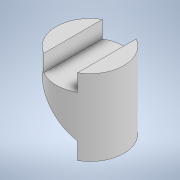
# Autodesk Inventor part: Деталь1вар2
Saved by Autodesk Inventor 2021.1 (Build 251245010, 245A)
## iProperties
Created: 2023-10-25
Part Number: Деталь1вар2
Material: Типовые
Document SubType Name: Modeling
Designer: Lenovo
Density: 1 g/cm^3
Appearance: По умолчанию
Author: Lenovo
Autodesk Inventor part; units mm, degrees
ref_plane "YZ Plane" through (0, 0, 0) normal (1, 0, 0) x (0, 1, 0)
ref_plane "XZ Plane" through (0, 0, 0) normal (0, 1, 0) x (-1, 0, 0)
ref_plane "XY Plane" through (0, 0, 0) normal (0, 0, 1) x (1, 0, 0)
sketch "Эскиз1" plane through (0, 0, 0) normal (0, 1, 0) x (-1, 0, 0)
  circle A0 centre (0, 0) radius 40
  dimension "d0" = 80
  constraints: 1 centre point, 1 coincident
  measures "d0" diameter of A0
extrude "Выдавливание1" add sketch "Эскиз1" along normal blind 90
sketch "Эскиз2" plane through (0, 0, 0) normal (0, 0, 1) x (1, 0, 0)
  line L0 (0, 70) -> (-20, 70)
  line L1 (-20, 70) -> (-20, 90)
  line L2 (0, 70) -> (20, 70)
  line L3 (20, 70) -> (20, 90)
  line L4 (20, 0) -> (20, 20)
  line L5 (20, 20) -> (-40, 70)
  line L6 (-40, 70) -> (-40, 0)
  line L7 (20, 0) -> (-40, 0)
  line L8 (-40, 0) -> (20, 0)
  line L9 (-20, 90) -> (20, 90)
  point P0 (0, 0)
  constraints: 20 end point, 4 point on line, 1 perpendicular
extrude "Выдавливание2" cut sketch "Эскиз2" against normal mid plane 1000
